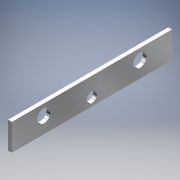
# Autodesk Inventor part: Inner Plate
Saved by Autodesk Inventor 2019.4 (Build 234330000, 330)
## iProperties
Created: 2019-12-07
Part Number: Inner Plate
Material: Aluminum 6061
Document SubType Name: Modeling
Designer: admin
Density: 2.7 g/cm^3
Appearance: Aluminum - Flat
Mass: 453.945 g
Surface Area: 568.361 cm^2
Volume: 168.128 cm^3
Author: admin
Autodesk Inventor part; units mm, degrees
ref_plane "YZ Plane" through (0, 0, 0) normal (1, 0, 0) x (0, 1, 0)
ref_plane "XZ Plane" through (0, 0, 0) normal (0, 1, 0) x (-1, 0, 0)
ref_plane "XY Plane" through (0, 0, 0) normal (0, 0, 1) x (1, 0, 0)
sketch "Sketch1" plane through (0, 0, 0) normal (1, 0, 0) x (0, 1, 0)
  line L0 (49.2406, -253.3994) -> (-0.7594, -253.3994)
  line L1 (-0.7594, -253.3994) -> (-0.7594, 46.6006)
  line L2 (-0.7594, 46.6006) -> (49.2406, 46.6006)
  line L3 (49.2406, 46.6006) -> (49.2406, -253.3994)
  circle A0 centre (29.2406, -193.3994) radius 12.5
  circle A1 centre (29.2406, -13.3994) radius 12.5
  line L4 (29.2406, -193.3994) -> (29.2406, -13.3994) construction
  line L5 (29.2406, -103.3994) -> (2.7957, -103.3994) construction
  point P0 (0, 0)
  dimension "d2" = 50
  dimension "d3" = 300
  dimension "d4" = 25
  dimension "d5" = 25
  dimension "d7" = 180
  dimension "d8" = 30
  dimension "d9" = 150
  constraints: 12 end point, 2 centre point, 2 horizontal, 2 parallel, 1 midpoint, 1 perpendicular, 1 vertical
  measures "d2" distance of L0.start L0.end
  measures "d3" distance of L2.end L0.start
  measures "d4" diameter of A0
  measures "d5" diameter of A1
  measures "d7" distance of L4.end L4.start
  measures "d8" distance between parallel lines of L1 L4
  measures "d9" distance between parallel lines of L0 L5
extrude "Extrusion1" add sketch "Sketch1" along normal blind 7
sketch "Sketch2" plane through (7, 0, 0) normal (1, 0, 0) x (0, 0, -1)
  line L0 (253.3994, 49.2406) -> (-46.6006, 49.2406) projected
  line L1 (103.3994, 49.2406) -> (103.3994, -0.7594) construction
  line L2 (-46.6006, -0.7594) -> (253.3994, -0.7594) projected
  circle A0 centre (103.3994, 14.2406) radius 9.5
  circle A1 centre (56.4094, 14.2406) radius 9.5
  circle A2 centre (150.3894, 14.2406) radius 9.5
  point P0 (0, 0)
  dimension "d10" = 19
  dimension "d11" = 35
  dimension "d14" = 19
  dimension "d15" = 19
  dimension "d16" = 35
  dimension "d17" = 35
  dimension "d18" = 46.99
  dimension "d19" = 46.99
  constraints: 3 centre point, 2 end point, 2 midpoint, 1 point on line
  measures "d10" diameter of A0
  measures "d11" distance from line of L0 A0.centre
  measures "d14" diameter of A1
  measures "d15" diameter of A2
  measures "d16" distance from line of L0 A2.centre
  measures "d17" distance from line of L0 A1.centre
  measures "d18" distance of A0.centre A1.centre
  measures "d19" distance of A0.centre A2.centre
extrude "Extrusion2" cut sketch "Sketch2" against normal blind 10
ref_plane "Work Plane1" through (0, 29.2406, 46.6006) normal (0, 1, 0) x (1, 0, 0)
equation "\"d9\" = 0.5 * d3"
body "Solid1"
